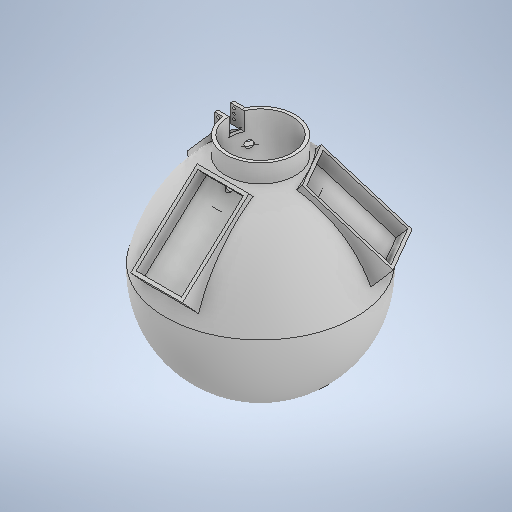
# Autodesk Inventor part: Water Sensor Bouy
Saved by Autodesk Inventor 2025 (Build 290162000, 162)
## iProperties
Created: 2024-06-17
Part Number: Water Sensor Bouy
Material: Generic
Document SubType Name: Modeling
Designer: track
Density: 1 g/cm^3
Appearance: Default
Mass: 1114.84 g
Surface Area: 2537.18 cm^2
Volume: 1114.84 cm^3
Author: track
## iProperties of the stored document Water Sensor Bouy_3DPrint.ipt
Created: 2024-06-17
Part Number: Water Sensor Bouy_3DPrint
Material: Generic
Document SubType Name: Modeling
Designer: track
Density: 1 g/cm^3
Appearance: Default
Author: track
Autodesk Inventor part; units mm, degrees
ref_plane "YZ Plane" through (0, 0, 0) normal (1, 0, 0) x (0, 1, 0)
ref_plane "XZ Plane" through (0, 0, 0) normal (0, 1, 0) x (-1, 0, 0)
ref_plane "XY Plane" through (0, 0, 0) normal (0, 0, 1) x (1, 0, 0)
sketch "Sketch1" plane through (0, 0, 0) normal (0, 0, 1) x (1, 0, 0)
  line L0 (0, 0) -> (0, 76.2)
  line L1 (25.3, 0) -> (25.3, 152.4)
  line L2 (25.3, 76.2) -> (76.1, 76.2)
  arc A0 (76.1, 76.2) -> (25.3, 152.4) centre (-47.8628, 48.5915) ccw
  arc A1 (25.3, 0) -> (76.1, 76.2) centre (0.0223, 71.8852) ccw
  line L3 (35.3, 130.8894) -> (35.3, 15.868)
  arc A2 (35.3, 15.868) -> (66.1566, 74.8322) centre (0.0223, 71.8852) ccw
  arc A3 (66.1566, 74.8322) -> (35.3, 130.8894) centre (-47.8628, 48.5915) ccw
  point P0 (25.3, 50.8)
  dimension "d1" = 25.3
  dimension "d3" = 0
  dimension "d74" = 152.4
  dimension "d75" = 50.8
  dimension "d76" = 76.2
  dimension "d78" = 127
  dimension "d83" = 10
  dimension "d128" = 83.1628
  dimension "d129" = 76.2
  constraints: 8 end point, 8 point on circle, 4 centre point, 2 vertical, 1 horizontal, 1 midpoint, 1 point on line, 2 other
  measures "d1" distance between parallel lines of L1 L0
  measures "d3" vertical distance of L0.start L1.start
  measures "d74" distance of L1.start L1.end
  measures "d75" distance of L2.start L2.end
  measures "d76" distance from line of L1.end L2
  measures "d78" radius of A0
  measures "d83" distance between parallel lines of L1 L3
  measures "d128" distance from line of L3 A0.centre
  measures "d129" radius of A1
revolve "Revolution1" add sketch "Sketch1" angle 360 about axis through (0, 0, 0) along (0, 1, 0) contours L1 L2 L3 A2 A3 A1 | L1 A0 L2 A3 L3
sketch "Sketch13" plane through (0, 0, 0) normal (0, 0, 1) x (1, 0, 0)
  line L0 (25.3, 152.4) -> (-25.3, 152.4) projected
  line L1 (0, 152.4) -> (0, 180.8136)
  line L2 (-25.3, 152.4) -> (-25.3, 165.1)
  line L3 (-25.3, 165.1) -> (-27.84, 165.1)
  line L4 (-27.84, 165.1) -> (-27.84, 150.5625)
  arc A0 (-25.3, 152.4) -> (-76.1, 76.2) centre (47.8628, 48.5915) ccw projected
  arc A1 (-25.3, 152.4) -> (-27.84, 150.5625) centre (47.8628, 48.5915) ccw
  point P0 (0, 0)
  dimension "d79" = 2.54
  dimension "d81" = 12.7
  constraints: 8 end point, 3 point on circle, 2 perpendicular, 2 vertical, 1 centre point, 1 concentric, 1 midpoint
  measures "d79" distance of L2.end L3.end
  measures "d81" distance of L0.end L2.end
revolve "Revolution2" add sketch "Sketch13" angle 350 about axis through (0, 152.4, 0) along (0, 1, 0)
sketch "Sketch17" plane through (0, 0, 0) normal (0, 0, 1) x (1, 0, 0)
  line L0 (-25.3, 152.4) -> (-25.3, 165.1) projected
  line L1 (-25.3, 165.1) -> (-34.19, 165.1)
  line L2 (-34.19, 165.1) -> (-34.19, 150.5625)
  line L3 (-34.19, 150.5625) -> (-25.3, 150.5625)
  line L4 (-25.3, 150.5625) -> (-25.3, 165.1)
  point P0 (0, 0)
  dimension "d91" = 8.89
  dimension "d92" = 14.5375
  constraints: 8 end point, 2 parallel, 1 horizontal, 1 perpendicular
  measures "d91" distance of L0.end L1.end
  measures "d92" distance of L1.end L2.end
extrude "Extrusion10" add sketch "Sketch17" along normal blind 2.54
sketch "Sketch18" plane through (-25.3, 152.4, 0) normal (0, 0, -1) x (-1, 0, 0)
  line L0 (0, 12.7) -> (8.89, 12.7) projected
  line L1 (0, 0) -> (0, 12.7) projected
  arc A0 (2.54, -1.8375) -> (0, 0) centre (-73.1628, -103.8085) ccw projected
  line L2 (8.89, -1.8375) -> (2.54, -1.8375) projected
  line L3 (8.89, 12.7) -> (8.89, -1.8375) projected
  line L4 (0, 0) -> (-0.3844, 0) projected
  arc A1 (50.8, -76.2) -> (0, 0) centre (-73.1628, -103.8085) ccw projected
  line L5 (0, 0) -> (2.54, -1.8375)
  line L6 (8.89, -1.8375) -> (2.54, -1.8375) projected
  line L7 (8.89, 12.7) -> (8.89, -1.8375) projected
  line L8 (8.89, -1.8375) -> (8.89, 12.7)
  line L9 (8.89, 12.7) -> (0, 12.7)
  point P0 (-25.3, -152.4)
  constraints: 6 end point, 1 perpendicular, 1 vertical
extrude "Extrusion11" add sketch "Sketch18" along normal blind 12.7 contours L0 L3 L2 A0 L1
sketch "Sketch20" plane through (-34.19, 150.5625, 2.54) normal (-1, 0, 0) x (0, 0, 1)
  line L0 (-15.24, 14.5375) -> (0, 14.5375) projected
  line L1 (-2.54, 0) -> (0, 0) projected
  line L2 (-12.7, 14.5375) -> (-2.54, 14.5375)
  line L3 (-2.54, 14.5375) -> (-2.54, 0)
  line L4 (-2.54, 0) -> (-12.7, 0)
  line L5 (-12.7, 0) -> (-12.7, 14.5375)
  line L6 (-15.24, 0) -> (-15.24, 14.5375) projected
  line L7 (0, 14.5375) -> (0, 0) projected
  point P0 (-2.54, -150.5625)
  point P1 (-2.54, 7.2687)
  point P2 (-2.54, 14.5375)
  dimension "d106" = 2.54
  dimension "d107" = 2.54
  constraints: 8 end point, 2 parallel, 2 point on line, 1 horizontal, 1 midpoint, 1 perpendicular
  measures "d106" distance between parallel lines of L6 L5
  measures "d107" distance from line of L7 point (-2.54, 7.269)
extrude "Extrusion12" cut sketch "Sketch20" against normal blind 17.78 contours L0 L3 L4 L5
sketch "Sketch21" plane through (0, 0, 2.54) normal (0, 0, 1) x (1, 0, 0)
  circle A0 centre (-31.5339, 162.56) radius 1
  circle A1 centre (-31.5339, 158.75) radius 1
  circle A2 centre (-31.5339, 154.94) radius 1
  line L0 (-31.5339, 162.56) -> (-31.5339, 154.94)
  line L1 (-31.5339, 154.94) -> (-27.7239, 154.94)
  line L2 (-27.7239, 165.1) -> (-27.7239, 150.5625) projected
  line L3 (-27.7239, 165.1) -> (-34.19, 165.1) projected
  point P0 (0, 0)
  dimension "d110" = 90
  dimension "d112" = 2
  dimension "d113" = 2
  dimension "d114" = 2
  dimension "d115" = 3.81
  dimension "d116" = 2.54
  dimension "d119" = 0
  dimension "d120" = 3.81
  dimension "d122" = 3.81
  constraints: 4 end point, 3 centre point, 1 horizontal, 1 midpoint, 1 point on line
  measures "d110" angle of L1 L0
  measures "d112" diameter of A0
  measures "d113" diameter of A1
  measures "d114" diameter of A2
  measures "d115" distance of L0.end L1.end
  measures "d116" distance from line of L3 L0.start
  measures "d119" distance from line of L0 A1.centre
  measures "d120" distance of L0.start A1.centre
  measures "d122" distance of point (-31.534, 158.75) L0.end
extrude "Extrusion13" cut sketch "Sketch21" against normal up to surface (15.24 mm away)
sketch "Sketch22" plane through (0, 0, 0) normal (1, 0, 0) x (0, 1, 0)
  arc A0 (150.5625, 27.84) -> (76.2, 76.1) centre (48.5915, -47.8628) ccw projected
  arc A1 (76.2, 76.1) -> (0, 25.3) centre (71.8852, 0.0223) ccw projected
  line L0 (142.0762, 38.1) -> (74.8322, -18.3245)
  line L1 (74.8322, -66.1566) -> (74.8322, 66.1566) projected
  line L2 (150.5625, 0) -> (165.1, 0) projected
  line L3 (74.8322, 0) -> (165.1, 0)
  point P0 (0, 0)
  dimension "d125" = 50
  dimension "d127" = 38.1
  constraints: 4 end point, 1 collinear, 1 midpoint, 1 point on circle, 1 point on line
  measures "d125" angle of L1 L0
  measures "d127" distance from line of L0.start L3
ref_plane "Work Plane6" through (0, 142.0762, 38.1) normal (0, 0.7361005, 0.6768723) x (-1, 0, 0)
sketch "Sketch23" plane through (0, 142.0762, 38.1) normal (0, 0.7361005, 0.6768723) x (-1, 0, 0)
  line L0 (18.25, -8.3895) -> (-18.25, -8.3895)
  line L1 (-18.25, -8.3895) -> (-18.25, 59.1105)
  line L2 (-18.25, 59.1105) -> (18.25, 59.1105)
  line L3 (18.25, 59.1105) -> (18.25, -8.3895)
  ellipse E0 centre (0, -33.7895) end of major axis (27.84, -33.7895) minor radius 20.493 (27.7239, -31.9198) -> (25.9199, -41.2683) ccw projected
  line L4 (-20.79, 61.6505) -> (-20.79, -10.9295)
  line L5 (-20.79, -10.9295) -> (20.79, -10.9295)
  line L6 (20.79, -10.9295) -> (20.79, 61.6505)
  line L7 (20.79, 61.6505) -> (-20.79, 61.6505)
  point P0 (0, 68.122)
  dimension "d130" = 36.5
  dimension "d131" = 67.5
  dimension "d132" = 25.4
  dimension "d133" = 18.25
  dimension "d134" = 2.54
  constraints: 16 end point, 4 parallel, 2 perpendicular, 1 horizontal, 4 other
  measures "d130" distance of L0.start L0.end
  measures "d131" distance of L0.end L1.end
  measures "d132" distance from line of point (0, -33.79) L0
  measures "d133" distance from line of point (0, -33.79) L1
  measures "d134" distance between parallel lines of L1 L4
extrude "Extrusion14" add sketch "Sketch23" against normal up to surface
sketch "Sketch24" plane through (0, 142.0762, 38.1) normal (0, 0.7361005, 0.6768723) x (-1, 0, 0)
  line L0 (18.25, -8.3895) -> (-18.25, -8.3895) projected
  line L1 (-18.25, -8.3895) -> (-18.25, 59.1105) projected
  line L2 (18.25, -8.3895) -> (-18.25, -8.3895)
  line L3 (-18.25, -8.3895) -> (-18.25, 59.1105)
  line L4 (-18.25, 59.1105) -> (18.25, 59.1105)
  line L5 (18.25, 59.1105) -> (18.25, -8.3895)
  point P0 (0, 68.122)
  constraints: 8 end point, 2 parallel, 1 horizontal, 1 perpendicular
extrude "Extrusion15" cut sketch "Sketch24" against normal blind 10
sketch "Sketch25" plane through (0, 0, 0) normal (0, 0, 1) x (1, 0, 0)
  circle A0 centre (0, 141.4049) radius 3
  line L0 (-18.25, 147.7549) -> (18.25, 147.7549) projected
  line L1 (18.25, 147.7549) -> (18.25, 102.066) projected
  point P0 (0, 0)
  dimension "d139" = 6
  dimension "d140" = 6.35
  dimension "d141" = 18.25
  constraints: 1 centre point
  measures "d139" diameter of A0
  measures "d140" distance from line of L0 A0.centre
  measures "d141" distance from line of L1 A0.centre
extrude "Extrusion16" cut sketch "Sketch25" along normal blind 63.5
sketch "Sketch26" plane through (0, 134.7152, 31.3313) normal (0, 0.7361005, 0.6768723) x (1, 0, 0)
  line L0 (-18.25, -59.1105) -> (-18.25, 8.3895) projected
  line L1 (18.25, 8.3895) -> (18.25, -59.1105) projected
  line L2 (-18.25, -33.7105) -> (18.25, -33.7105)
  line L3 (18.25, -33.7105) -> (18.25, -59.1105)
  line L4 (18.25, -59.1105) -> (-18.25, -59.1105)
  line L5 (-18.25, -59.1105) -> (-18.25, -33.7105)
  point P0 (0, -68.122)
  point P1 (-18.25, -59.1105)
  point P2 (18.25, -33.7105)
  dimension "d144" = 25.4
  constraints: 8 end point, 2 parallel, 1 horizontal, 1 perpendicular, 1 point on line
  measures "d144" distance between parallel lines of L4 L2
extrude "Extrusion17" add sketch "Sketch26" against normal blind 10
pattern_circular "Circular Pattern4" count 3 over 360 about axis through (0, 157.8313, 0) along (0, 1, 0) of "Extrusion14", "Extrusion15", "Extrusion16", "Extrusion17"
sketch "Sketch27" plane through (0, 0, 0) normal (0, 1, 0) x (-1, 0, 0)
  line L0 (0, 0) -> (-76.1, 0)
  circle A0 centre (0, 0) radius 76.1 projected
  circle A1 centre (-50.8, 0) radius 3.175
  dimension "d150" = 6.35
  dimension "d151" = 50.8
  constraints: 2 end point, 1 centre point, 1 horizontal, 1 horizontal alignment, 1 point on line, 1 other
  measures "d150" diameter of A1
  measures "d151" distance of L0.start A1.centre
extrude "Extrusion18" cut sketch "Sketch27" along normal blind 33.02 contours A1 L0 | L0 A1
pattern_circular "Circular Pattern5" count 3 over 360 about axis through (0, 71.8852, 0) along (0, 1, 0) of "Extrusion18"
body "Solid1"
